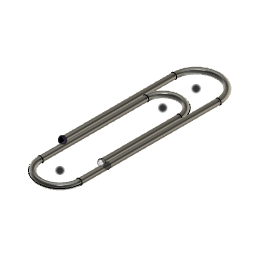
Semana2_Desafio5 (Autodesk Fusion 360 design; units mm, degrees)
Autodesk Fusion 360 part; units mm, degrees
sketch "Sketch1" plane through (0, 0, 0) normal (0, 0, 1) x (1, 0, 0)
  line L0 (0, 0) -> (0, 20)
  line L1 (1, 13.9967) -> (1, -5)
  line L2 (8, 20) -> (8, -5)
  arc A0 (7, 13.9967) -> (1, 13.9967) centre (4, 13.9967) ccw
  line L3 (7, 13.9967) -> (7, 0)
  arc A1 (8, 20) -> (0, 20) centre (4, 20) ccw
  arc A2 (1, -5) -> (8, -5) centre (4.5, -5) ccw
  point P0 (8, 0)
  dimension "d3" = 25
  dimension "d4" = 20
  dimension "d24" = 8
  dimension "d25" = 6
  dimension "d27" = 7
  dimension "d28" = 5
  dimension "d29" = 6.0033
  dimension "d30" = 5
  constraint coincident L0.start origin
  constraint vertical L0
  constraint parallel L0 L1
  constraint parallel L1 L2
  constraint tangent L1 A0
  constraint tangent A0 L3
  constraint vertical L3
  constraint coincident L2 P0
  constraint horizontal L0.start P0
  constraint tangent L0 A1
  constraint tangent L1 A2
  measures "d3" distance of L2.start L2.end
  measures "d4" distance of L0.start L0.end
  measures "d24" distance of L0 L2
  measures "d25" distance of L1 L3
  measures "d27" distance of L1 L2
  measures "d28" distance of L2.end P0
  measures "d29" distance of A0.centre A1.centre
  measures "d30" vertical distance of L0.start A2.centre
sketch "Sketch2" plane through (0, 0, 0) normal (0, 1, 0) x (1, 0, 0)
  circle A0 centre (0, 0) radius 0.5
  dimension "d7" = 1
  constraint coincident A0.centre origin
  measures "d7" diameter of A0
sweep "Sweep3" add profiles "Sketch2" path "Sketch1" along L3 A0 L1 A2 L2 A1 L0 section 1
